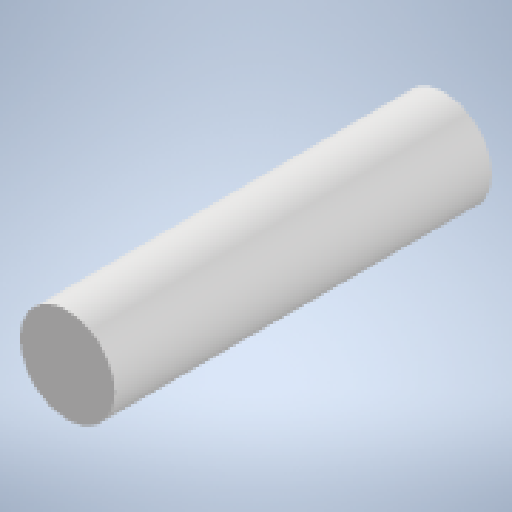
# Autodesk Inventor part: MotorPart3
Saved by Autodesk Inventor 2024 (Build 280153000, 153)
## iProperties
Created: 2024-10-17
Part Number: MotorPart3
Material: 一般
Document SubType Name: Modeling
Designer: jerry
Density: 1 g/cm^3
Appearance: 預設
Author: jerry
Autodesk Inventor part; units mm, degrees
ref_plane "YZ Plane" through (0, 0, 0) normal (1, 0, 0) x (0, 1, 0)
ref_plane "XZ Plane" through (0, 0, 0) normal (0, 1, 0) x (-1, 0, 0)
ref_plane "XY Plane" through (0, 0, 0) normal (0, 0, 1) x (1, 0, 0)
sketch "草圖1" plane through (0, 0, 0) normal (0, 0, 1) x (1, 0, 0)
  circle A0 centre (0, 0) radius 5
  dimension "d0" = 10
  constraints: 1 centre point, 1 coincident
  measures "d0" diameter of A0
extrude "擠出1" add sketch "草圖1" along normal blind 40
sketch "草圖2" plane through (0, 0, 40) normal (0, 0, 1) x (1, 0, 0)
  circle A0 centre (0, 0) radius 2.5
  circle A1 centre (0, 0) radius 5 projected
  line L0 (-4.3301, -7.5) -> (4.3301, -7.5)
  line L1 (4.3301, -7.5) -> (4.3301, -2.5)
  line L2 (4.3301, -2.5) -> (-4.3301, -2.5)
  line L3 (-4.3301, -2.5) -> (-4.3301, -7.5)
  line L4 (-4.3301, -7.5) -> (4.3301, -2.5) construction
  line L5 (4.3301, -7.5) -> (-4.3301, -2.5) construction
  point P0 (0, -5)
  dimension "d3" = 5
  constraints: 12 end point, 2 midpoint, 2 parallel, 2 point on circle, 1 centre point, 1 coincident, 1 horizontal, 1 perpendicular
  measures "d3" diameter of A0
extrude "擠出2" cut sketch "草圖2" against normal blind 10 contours L2 A1 picked at (-2.6557, -2.8104)
